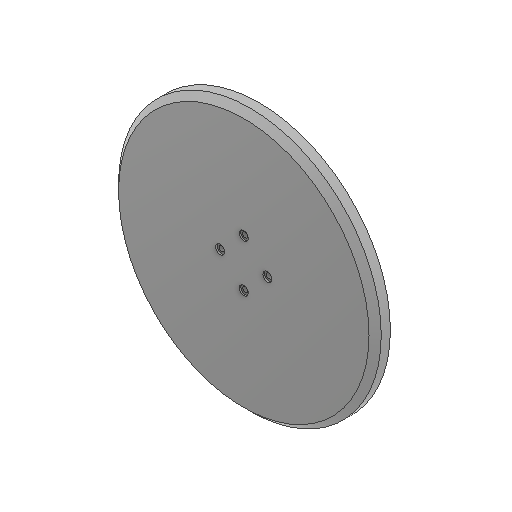
# Autodesk Inventor part: hoverboardHubCap
Saved by Autodesk Inventor 2025 (Build 290162000, 162)
## iProperties
Created: 2024-12-05
Part Number: hoverboardHubCap
Material: ABS Plastic
Document SubType Name: Modeling
Designer: derm
Density: 1.06 g/cm^3
Appearance: Smooth - Medium Gray
Author: derm
Autodesk Inventor part; units mm, degrees
ref_plane "YZ Plane" through (0, 0, 0) normal (1, 0, 0) x (0, 1, 0)
ref_plane "XZ Plane" through (0, 0, 0) normal (0, 1, 0) x (-1, 0, 0)
ref_plane "XY Plane" through (0, 0, 0) normal (0, 0, 1) x (1, 0, 0)
sketch "Sketch1" plane through (0, 0, 0) normal (0, 0, 1) x (1, 0, 0)
  circle A0 centre (0, 0) radius 69
  dimension "d0" = 138
  constraints: 1 centre point, 1 coincident
  measures "d0" diameter of A0
extrude "Extrusion1" add sketch "Sketch1" against normal blind 6
sketch "Sketch2" plane through (0, 0, 0) normal (0, 0, 1) x (1, 0, 0)
  circle A0 centre (0, 0) radius 86.0347
  constraints: 1 centre point, 1 coincident
extrude "Extrusion2" add sketch "Sketch2" along normal blind 10
sketch "Sketch3" plane through (0, 0, 10) normal (0, 0, 1) x (1, 0, 0)
  circle A0 centre (0, 0) radius 86.0347 projected
  circle A1 centre (0, 0) radius 15.5 construction
  circle A2 centre (0, 15.5) radius 1.75
  circle A3 centre (-15.5, 0) radius 1.75
  circle A4 centre (0, -15.5) radius 1.75
  circle A5 centre (15.5, 0) radius 1.75
  dimension "d5" = 31
  dimension "d6" = 3.5
  dimension "d9" = 360
  constraints: 4 centre point, 1 coincident, 1 vertical alignment, 11 other
  measures "d6" diameter of A2
extrude "Extrusion3" cut sketch "Sketch3" against normal through all contours A2 | A3 | A4 | A5
sketch "Sketch4" plane through (0, 0, 10) normal (0, 0, 1) x (1, 0, 0)
  circle A0 centre (15.5, 0) radius 1.75 projected
  circle A1 centre (-15.5, 0) radius 1.75 projected
  circle A2 centre (0, -15.5) radius 1.75 projected
  circle A3 centre (0, 15.5) radius 1.75 projected
  circle A4 centre (0, 0) radius 86.0347 projected
  circle A5 centre (0, -15.5) radius 3
  circle A6 centre (15.5, 0) radius 3
  circle A7 centre (0, 15.5) radius 3
  circle A8 centre (-15.5, 0) radius 3
  dimension "d13" = 6
  dimension "d16" = 360
  constraints: 4 centre point, 1 coincident, 9 other
  measures "d13" diameter of A5
extrude "Extrusion4" cut sketch "Sketch4" against normal blind 1 contours A0 | A1 | A3 | A5 | A6 | A7 | A8
sketch "Sketch5" plane through (0, 0, 0) normal (1, 0, 0) x (0, 1, 0)
  line L0 (86.0347, 10) -> (-86.0347, 10) projected
  line L1 (-86.0347, 0) -> (-86.0347, 10) projected
  line L2 (0, 0) -> (0, 58.0565)
  line L3 (-22.0852, 10) -> (-23.5623, 10) construction
  line L4 (-23.5623, 10) -> (-67.5613, 8.2465) construction
  line L5 (-67.5613, 8.2465) -> (-86.0347, 1.135) construction
  spline S0 degree 3 poles (-22.0852, 10) (-23.5623, 10) (-67.5613, 8.2465) (-86.0347, 1.135) knots 1 1 1 1 2 2 2 2
  constraints: 2 end point, 2 point on line, 1 vertical, 3 other
revolve "Revolution1" [suppressed]
sketch "Sketch6" plane through (0, 0, -6) normal (0, 0, -1) x (-1, 0, 0)
  circle A0 centre (-15.5, 0) radius 1.75 projected
  circle A1 centre (15.5, 0) radius 1.75 projected
  circle A2 centre (0, -15.5) radius 1.75 projected
  circle A3 centre (0, 15.5) radius 1.75 projected
  circle A4 centre (0, 0) radius 69 projected
  circle A5 centre (0, 0) radius 64.6782
  constraints: 1 centre point, 1 coincident
extrude "Extrusion5" cut sketch "Sketch6" against normal blind 8 contours A5
chamfer "Chamfer1" distance 4 angle 45 1 edges at (-86.0347, 0, 10)
chamfer "Chamfer2" distance 2 angle 45 1 edges at (64.6782, 0, -6)
sketch "Sketch7" plane through (0, 0, 2) normal (0, 0, -1) x (-1, 0, 0)
  circle A0 centre (0, 0) radius 64.6782 projected
  circle A1 centre (0, 15.5) radius 1.75 projected
  circle A2 centre (0, -15.5) radius 1.75 projected
  circle A3 centre (15.5, 0) radius 1.75 projected
  circle A4 centre (-15.5, 0) radius 1.75 projected
extrude "Extrusion6" cut sketch "Sketch7" against normal blind 3
body "Solid1"
